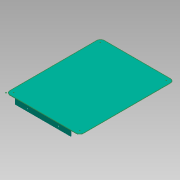
# Autodesk Inventor part: Cart_TOP_SHELF
Saved by Autodesk Inventor 2015 (Build 190159000, 159)
## iProperties
Created: 2015-05-21
Part Number: Cart_TOP_SHELF
Material: Cart Material
Document SubType Name: Modeling
Designer: Joe Sheldon
Density: 1 g/cm^3
Appearance: Default
Author: Joe Sheldon
Autodesk Inventor part; units mm, degrees
ref_plane "YZ Plane" through (0, 0, 0) normal (1, 0, 0) x (0, 1, 0)
ref_plane "XZ Plane" through (0, 0, 0) normal (0, 1, 0) x (-1, 0, 0)
ref_plane "XY Plane" through (0, 0, 0) normal (0, 0, 1) x (1, 0, 0)
sketch "Sketch1" plane through (0, 0, 0) normal (0, 1, 0) x (-1, 0, 0)
  line L0 (0, 0) -> (-361.95, 0)
  line L1 (-361.95, 0) -> (-361.95, -463.55)
  line L2 (-361.95, -463.55) -> (0, -463.55)
  line L3 (0, -463.55) -> (0, 0)
  dimension "d0" = 361.95
  dimension "d1" = 463.55
  constraints: 8 end point, 2 parallel, 1 horizontal, 1 perpendicular
  measures "d0" distance of L2.end L1.end
  measures "d1" distance of L1.end L0.end
extrude "Extrusion1" add sketch "Sketch1" along normal blind 2.794
fillet "Fillet1" radius 19.05 4 edges at (361.95, 1.397, 0) (361.95, 1.397, -463.55) (0, 1.397, -463.55) (0, 1.397, 0)
sketch "Sketch2" plane through (0, 0, 0) normal (0, -1, 0) x (1, 0, 0)
  line L0 (19.05, 0) -> (342.9, 0)
  line L1 (342.9, 0) -> (342.9, -2.8525)
  line L2 (342.9, -2.8525) -> (19.05, -2.8525)
  line L3 (19.05, -2.8525) -> (19.05, 0)
  line L4 (342.9, -2.8525) -> (317.5, -2.8525)
  line L5 (317.5, -2.8525) -> (317.5, 0)
  line L6 (317.5, 0) -> (342.9, 0)
  line L7 (342.9, 0) -> (342.9, -2.8525)
  line L8 (19.05, -2.8525) -> (44.45, -2.8525)
  line L9 (44.45, -2.8525) -> (44.45, 0)
  line L10 (44.45, 0) -> (19.05, 0)
  line L11 (19.05, 0) -> (19.05, -2.8525)
  line L12 (44.45, -2.8525) -> (317.5, -2.8525)
  line L13 (317.5, -2.8525) -> (317.5, 0)
  line L14 (317.5, 0) -> (44.45, 0)
  line L15 (44.45, 0) -> (44.45, -2.8525)
  point P0 (0, 0)
  dimension "d5" = 25.4
  dimension "d6" = 25.4
  constraints: 32 end point, 8 parallel, 4 horizontal, 4 perpendicular, 2 point on line
  measures "d5" distance of L5.end L6.end
  measures "d6" distance of L10.end L9.end
extrude "Extrusion2" add sketch "Sketch2" along normal blind 25.4 contours L0 L5 L2 L9
sketch "Sketch3" plane through (19.05, 2.794, 0) normal (0, 0, 1) x (1, 0, 0)
  line L0 (323.85, -2.794) -> (0, -2.794) projected
  line L1 (25.405, -2.794) -> (25.4, -15.494)
  line L2 (25.4, -2.794) -> (25.4, -28.194) projected
  line L3 (25.4, -15.494) -> (85.4, -15.5178)
  line L4 (298.45, -2.794) -> (298.45, -28.194) projected
  line L5 (298.45, -15.494) -> (238.45, -15.494)
  circle A0 centre (85.4, -15.5178) radius 3.429
  circle A1 centre (238.45, -15.494) radius 3.429
  point P0 (-19.05, -2.794)
  dimension "d9" = 12.7
  dimension "d10" = 60
  dimension "d11" = 60
  dimension "d12" = 6.858
  dimension "d13" = 6.858
  constraints: 6 end point, 2 centre point, 2 coincident, 2 midpoint, 1 horizontal, 1 perpendicular, 1 point on line
  measures "d9" distance of L1.start L1.end
  measures "d10" distance of L1.end L3.end
  measures "d11" distance of L5.start L5.end
  measures "d12" diameter of A0
  measures "d13" diameter of A1
extrude "Extrusion3" cut sketch "Sketch3" against normal blind 25.4 contours A0 | A1
sketch "Sketch4" plane through (0, 2.794, 0) normal (0, 1, 0) x (1, 0, 0)
  arc A0 (0, 19.05) -> (19.05, 0) centre (19.05, 19.05) ccw projected
  line L0 (19.05, 0) -> (342.9, 0) projected
  arc A1 (342.9, 0) -> (361.95, 19.05) centre (342.9, 19.05) ccw projected
  line L1 (361.95, 19.05) -> (361.95, 444.5) projected
  arc A2 (361.95, 444.5) -> (342.9, 463.55) centre (342.9, 444.5) ccw projected
  line L2 (342.9, 463.55) -> (19.05, 463.55) projected
  arc A3 (19.05, 463.55) -> (0, 444.5) centre (19.05, 444.5) ccw projected
  line L3 (0, 444.5) -> (0, 19.05) projected
  point P0 (0, 0)
body "Solid1"
